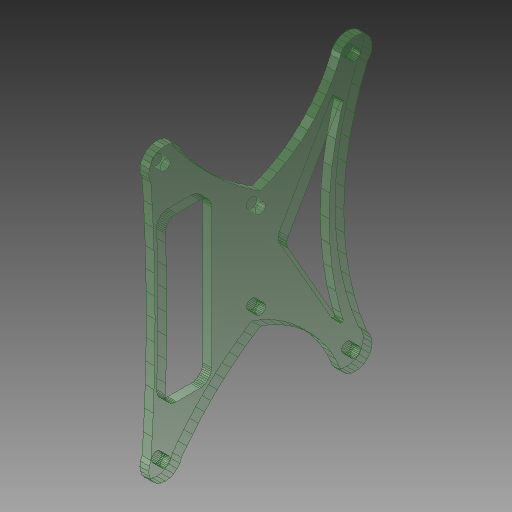
# Autodesk Inventor part: LCD Back
Saved by Autodesk Inventor 2017 (Build 210142000, 142)
## iProperties
Created: 2016-07-27
Part Number: LCD Back
Material: Polycarbonate, Green
Document SubType Name: Modeling
Designer: User
Density: 1.2 g/cm^3
Appearance: Polycarbonate - Clear(2)
Author: User
Autodesk Inventor part; units mm, degrees
ref_plane "YZ Plane" through (0, 0, 0) normal (1, 0, 0) x (0, 1, 0)
ref_plane "XZ Plane" through (0, 0, 0) normal (0, 1, 0) x (-1, 0, 0)
ref_plane "XY Plane" through (0, 0, 0) normal (0, 0, 1) x (1, 0, 0)
sketch "Sketch1" plane through (0, 0, 0) normal (1, 0, 0) x (0, 1, 0)
  line L0 (99.8582, 85.8976) -> (98.9523, 87.0781)
  line L1 (98.9523, 87.0781) -> (97.7718, 87.984)
  line L2 (97.7718, 87.984) -> (96.3971, 88.5535)
  line L3 (96.3971, 88.5535) -> (93.4934, 89.8678)
  line L4 (93.4934, 89.8678) -> (90.6898, 91.384)
  line L5 (90.6898, 91.384) -> (88.0005, 93.0948)
  line L6 (88.0005, 93.0948) -> (85.4388, 94.9914)
  line L7 (85.4388, 94.9914) -> (83.0176, 97.0643)
  line L8 (83.0176, 97.0643) -> (80.7493, 99.3035)
  line L9 (80.7493, 99.3035) -> (78.645, 101.6974)
  line L10 (78.645, 101.6974) -> (76.7151, 104.2342)
  line L11 (76.7151, 104.2342) -> (74.9695, 106.901)
  line L12 (74.9695, 106.901) -> (73.4169, 109.6846)
  line L13 (73.4169, 109.6846) -> (72.0648, 112.571)
  line L14 (72.0648, 112.571) -> (70.9203, 115.5457)
  line L15 (70.9203, 115.5457) -> (72.6238, 118.1505)
  line L16 (72.6238, 118.1505) -> (74.4103, 120.699)
  line L17 (74.4103, 120.699) -> (76.2779, 123.1886)
  line L18 (76.2779, 123.1886) -> (78.2249, 125.6168)
  line L19 (78.2249, 125.6168) -> (80.2491, 127.9809)
  line L20 (80.2491, 127.9809) -> (82.3484, 130.2786)
  line L21 (82.3484, 130.2786) -> (84.5207, 132.5074)
  line L22 (84.5207, 132.5074) -> (86.7637, 134.6651)
  line L23 (86.7637, 134.6651) -> (89.075, 136.7494)
  line L24 (89.075, 136.7494) -> (91.4523, 138.7582)
  line L25 (91.4523, 138.7582) -> (93.8931, 140.6893)
  line L26 (93.8931, 140.6893) -> (96.394, 142.5437)
  line L27 (96.394, 142.5437) -> (97.7687, 143.1132)
  line L28 (97.7687, 143.1132) -> (98.9492, 144.0191)
  line L29 (98.9492, 144.0191) -> (99.8551, 145.1995)
  line L30 (99.8551, 145.1995) -> (100.4246, 146.5743)
  line L31 (100.4246, 146.5743) -> (100.6188, 148.0495)
  line L32 (100.6188, 148.0495) -> (100.4246, 149.5241)
  line L33 (100.4246, 149.5241) -> (99.8552, 150.8989)
  line L34 (99.8552, 150.8989) -> (98.9493, 152.0793)
  line L35 (98.9493, 152.0793) -> (97.7688, 152.9852)
  line L36 (97.7688, 152.9852) -> (96.3941, 153.5547)
  line L37 (96.3941, 153.5547) -> (94.9188, 153.7489)
  line L38 (94.9188, 153.7489) -> (93.4436, 153.5547)
  line L39 (93.4436, 153.5547) -> (93.2768, 153.4856)
  line L40 (93.2768, 153.4856) -> (92.0689, 152.9852)
  line L41 (92.0689, 152.9852) -> (85.2186, 152.5575)
  line L42 (85.2186, 152.5575) -> (78.3639, 152.2075)
  line L43 (78.3639, 152.2075) -> (71.5057, 151.9352)
  line L44 (71.5057, 151.9352) -> (64.6449, 151.7407)
  line L45 (64.6449, 151.7407) -> (57.7823, 151.624)
  line L46 (57.7823, 151.624) -> (50.9188, 151.5851)
  line L47 (50.9188, 151.5851) -> (44.0554, 151.624)
  line L48 (44.0554, 151.624) -> (37.1928, 151.7407)
  line L49 (37.1928, 151.7407) -> (30.332, 151.9352)
  line L50 (30.332, 151.9352) -> (23.4738, 152.2077)
  line L51 (23.4738, 152.2077) -> (16.6191, 152.5579)
  line L52 (16.6191, 152.5579) -> (9.7689, 152.9858)
  line L53 (9.7689, 152.9858) -> (8.3942, 153.5553)
  line L54 (8.3942, 153.5553) -> (6.9189, 153.7495)
  line L55 (6.9189, 153.7495) -> (5.4436, 153.5553)
  line L56 (5.4436, 153.5553) -> (4.0689, 152.9858)
  line L57 (4.0689, 152.9858) -> (2.8885, 152.0799)
  line L58 (2.8885, 152.0799) -> (1.9826, 150.8995)
  line L59 (1.9826, 150.8995) -> (1.4131, 149.5248)
  line L60 (1.4131, 149.5248) -> (1.2189, 148.0495)
  line L61 (1.2189, 148.0495) -> (1.4131, 146.5742)
  line L62 (1.4131, 146.5742) -> (1.9825, 145.1995)
  line L63 (1.9825, 145.1995) -> (2.8884, 144.019)
  line L64 (2.8884, 144.019) -> (4.0689, 143.1131)
  line L65 (4.0689, 143.1131) -> (5.4436, 142.5436)
  line L66 (5.4436, 142.5436) -> (7.9456, 140.6925)
  line L67 (7.9456, 140.6925) -> (10.3866, 138.7617)
  line L68 (10.3866, 138.7617) -> (12.7641, 136.7533)
  line L69 (12.7641, 136.7533) -> (15.0757, 134.6693)
  line L70 (15.0757, 134.6693) -> (17.3189, 132.5118)
  line L71 (17.3189, 132.5118) -> (19.4915, 130.2833)
  line L72 (19.4915, 130.2833) -> (21.5911, 127.9858)
  line L73 (21.5911, 127.9858) -> (23.6155, 125.6219)
  line L74 (23.6155, 125.6219) -> (25.5628, 123.194)
  line L75 (25.5628, 123.194) -> (27.4308, 120.7046)
  line L76 (27.4308, 120.7046) -> (29.2176, 118.1563)
  line L77 (29.2176, 118.1563) -> (30.9214, 115.5518)
  line L78 (30.9214, 115.5518) -> (29.7772, 112.5769)
  line L79 (29.7772, 112.5769) -> (28.4256, 109.6903)
  line L80 (28.4256, 109.6903) -> (26.8732, 106.9066)
  line L81 (26.8732, 106.9066) -> (25.1279, 104.2395)
  line L82 (25.1279, 104.2395) -> (23.1984, 101.7025)
  line L83 (23.1984, 101.7025) -> (21.0943, 99.3084)
  line L84 (21.0943, 99.3084) -> (18.8263, 97.0689)
  line L85 (18.8263, 97.0689) -> (16.4054, 94.9957)
  line L86 (16.4054, 94.9957) -> (13.8439, 93.0988)
  line L87 (13.8439, 93.0988) -> (11.1548, 91.3877)
  line L88 (11.1548, 91.3877) -> (8.3514, 89.8711)
  line L89 (8.3514, 89.8711) -> (5.4478, 88.5565)
  line L90 (5.4478, 88.5565) -> (4.0731, 87.987)
  line L91 (4.0731, 87.987) -> (2.8926, 87.0811)
  line L92 (2.8926, 87.0811) -> (1.9867, 85.9006)
  line L93 (1.9867, 85.9006) -> (1.4172, 84.5259)
  line L94 (1.4172, 84.5259) -> (1.223, 83.0507)
  line L95 (1.223, 83.0507) -> (1.4172, 81.5754)
  line L96 (1.4172, 81.5754) -> (1.9867, 80.2007)
  line L97 (1.9867, 80.2007) -> (2.8926, 79.0202)
  line L98 (2.8926, 79.0202) -> (4.0731, 78.1143)
  line L99 (4.0731, 78.1143) -> (5.4478, 77.5448)
  line L100 (5.4478, 77.5448) -> (6.923, 77.3506)
  line L101 (6.923, 77.3506) -> (8.3983, 77.5448)
  line L102 (8.3983, 77.5448) -> (9.773, 78.1143)
  line L103 (9.773, 78.1143) -> (11.0884, 79.0713)
  line L104 (11.0884, 79.0713) -> (17.3468, 81.4425)
  line L105 (17.3468, 81.4425) -> (22.6145, 83.0508)
  line L106 (22.6145, 83.0508) -> (23.8857, 83.4389)
  line L107 (23.8857, 83.4389) -> (30.5418, 85.0007)
  line L108 (30.5418, 85.0007) -> (37.2863, 86.1211)
  line L109 (37.2863, 86.1211) -> (44.0898, 86.7953)
  line L110 (44.0898, 86.7953) -> (50.9229, 87.0204)
  line L111 (50.9229, 87.0204) -> (57.7561, 86.7954)
  line L112 (57.7561, 86.7954) -> (64.5596, 86.1212)
  line L113 (64.5596, 86.1212) -> (71.3041, 85.0009)
  line L114 (71.3041, 85.0009) -> (77.9602, 83.4392)
  line L115 (77.9602, 83.4392) -> (79.2314, 83.0511)
  line L116 (79.2314, 83.0511) -> (84.4991, 81.4428)
  line L117 (84.4991, 81.4428) -> (90.7575, 79.0716)
  line L118 (90.7575, 79.0716) -> (90.8924, 79.0205)
  line L119 (90.8924, 79.0205) -> (92.0729, 78.1146)
  line L120 (92.0729, 78.1146) -> (93.4476, 77.5451)
  line L121 (93.4476, 77.5451) -> (94.9229, 77.3509)
  line L122 (94.9229, 77.3509) -> (96.3981, 77.5451)
  line L123 (96.3981, 77.5451) -> (97.7729, 78.1146)
  line L124 (97.7729, 78.1146) -> (98.9533, 79.0205)
  line L125 (98.9533, 79.0205) -> (99.858, 80.1993)
  line L126 (99.858, 80.1993) -> (100.4275, 81.574)
  line L127 (100.4275, 81.574) -> (100.6217, 83.0492)
  line L128 (100.6217, 83.0492) -> (100.4277, 84.5229)
  line L129 (100.4277, 84.5229) -> (99.8582, 85.8976)
  line L130 (96.5664, 148.4895) -> (96.3966, 148.8995)
  line L131 (96.3966, 148.8995) -> (96.1264, 149.2515)
  line L132 (96.1264, 149.2515) -> (95.7743, 149.5217)
  line L133 (95.7743, 149.5217) -> (95.3643, 149.6915)
  line L134 (95.3643, 149.6915) -> (94.9243, 149.7495)
  line L135 (94.9243, 149.7495) -> (94.4843, 149.6916)
  line L136 (94.4843, 149.6916) -> (94.0743, 149.5217)
  line L137 (94.0743, 149.5217) -> (93.7223, 149.2515)
  line L138 (93.7223, 149.2515) -> (93.4521, 148.8995)
  line L139 (93.4521, 148.8995) -> (93.2822, 148.4895)
  line L140 (93.2822, 148.4895) -> (93.2243, 148.0495)
  line L141 (93.2243, 148.0495) -> (93.2822, 147.6095)
  line L142 (93.2822, 147.6095) -> (93.3265, 147.5026)
  line L143 (93.3265, 147.5026) -> (93.4521, 147.1995)
  line L144 (93.4521, 147.1995) -> (93.7223, 146.8474)
  line L145 (93.7223, 146.8474) -> (94.0744, 146.5772)
  line L146 (94.0744, 146.5772) -> (94.4843, 146.4074)
  line L147 (94.4843, 146.4074) -> (94.9243, 146.3494)
  line L148 (94.9243, 146.3494) -> (95.3643, 146.4074)
  line L149 (95.3643, 146.4074) -> (95.7743, 146.5772)
  line L150 (95.7743, 146.5772) -> (96.1264, 146.8474)
  line L151 (96.1264, 146.8474) -> (96.3966, 147.1995)
  line L152 (96.3966, 147.1995) -> (96.5664, 147.6094)
  line L153 (96.5664, 147.6094) -> (96.6243, 148.0494)
  line L154 (96.6243, 148.0494) -> (96.5664, 148.4895)
  line L155 (78.5162, 144.7192) -> (78.4132, 145.2247)
  line L156 (78.4132, 145.2247) -> (78.2435, 145.7119)
  line L157 (78.2435, 145.7119) -> (78.0103, 146.1721)
  line L158 (78.0103, 146.1721) -> (77.7176, 146.597)
  line L159 (77.7176, 146.597) -> (77.3708, 146.9789)
  line L160 (77.3708, 146.9789) -> (76.9761, 147.3111)
  line L161 (76.9761, 147.3111) -> (76.5405, 147.5875)
  line L162 (76.5405, 147.5875) -> (76.0719, 147.8033)
  line L163 (76.0719, 147.8033) -> (75.5786, 147.9545)
  line L164 (75.5786, 147.9545) -> (75.0696, 148.0384)
  line L165 (75.0696, 148.0384) -> (74.5539, 148.0536)
  line L166 (74.5539, 148.0536) -> (71.6473, 147.9381)
  line L167 (71.6473, 147.9381) -> (64.7411, 147.7424)
  line L168 (64.7411, 147.7424) -> (57.8332, 147.6249)
  line L169 (57.8332, 147.6249) -> (50.9243, 147.5857)
  line L170 (50.9243, 147.5857) -> (44.0155, 147.6249)
  line L171 (44.0155, 147.6249) -> (37.1076, 147.7424)
  line L172 (37.1076, 147.7424) -> (30.2014, 147.9381)
  line L173 (30.2014, 147.9381) -> (26.8482, 148.0682)
  line L174 (26.8482, 148.0682) -> (26.3322, 148.0522)
  line L175 (26.3322, 148.0522) -> (25.8229, 147.9675)
  line L176 (25.8229, 147.9675) -> (25.3295, 147.8156)
  line L177 (25.3295, 147.8156) -> (24.8608, 147.5991)
  line L178 (24.8608, 147.5991) -> (24.4251, 147.322)
  line L179 (24.4251, 147.322) -> (24.0305, 146.9893)
  line L180 (24.0305, 146.9893) -> (23.6837, 146.6068)
  line L181 (23.6837, 146.6068) -> (23.3911, 146.1814)
  line L182 (23.3911, 146.1814) -> (23.1579, 145.7208)
  line L183 (23.1579, 145.7208) -> (22.9883, 145.2332)
  line L184 (22.9883, 145.2332) -> (22.8853, 144.7273)
  line L185 (22.8853, 144.7273) -> (22.8508, 144.2122)
  line L186 (22.8508, 144.2122) -> (22.8508, 136.3352)
  line L187 (22.8508, 136.3352) -> (22.8847, 135.8071)
  line L188 (22.8847, 135.8071) -> (22.986, 135.2877)
  line L189 (22.986, 135.2877) -> (23.1529, 134.7855)
  line L190 (23.1529, 134.7855) -> (23.3828, 134.3089)
  line L191 (23.3828, 134.3089) -> (23.6717, 133.8656)
  line L192 (23.6717, 133.8656) -> (24.0151, 133.463)
  line L193 (24.0151, 133.463) -> (24.4072, 133.1076)
  line L194 (24.4072, 133.1076) -> (24.8415, 132.8053)
  line L195 (24.8415, 132.8053) -> (25.311, 132.5611)
  line L196 (25.311, 132.5611) -> (25.8079, 132.3791)
  line L197 (25.8079, 132.3791) -> (26.324, 132.2621)
  line L198 (26.324, 132.2621) -> (26.8508, 132.2122)
  line L199 (26.8508, 132.2122) -> (74.5507, 132.2122)
  line L200 (74.5507, 132.2122) -> (75.0729, 132.2464)
  line L201 (75.0729, 132.2464) -> (75.586, 132.3485)
  line L202 (75.586, 132.3485) -> (76.0815, 132.5167)
  line L203 (76.0815, 132.5167) -> (76.5507, 132.7482)
  line L204 (76.5507, 132.7482) -> (76.9858, 133.0389)
  line L205 (76.9858, 133.0389) -> (77.3791, 133.3839)
  line L206 (77.3791, 133.3839) -> (77.7242, 133.7772)
  line L207 (77.7242, 133.7772) -> (78.0149, 134.2122)
  line L208 (78.0149, 134.2122) -> (78.2463, 134.6815)
  line L209 (78.2463, 134.6815) -> (78.4146, 135.177)
  line L210 (78.4146, 135.177) -> (78.5167, 135.6901)
  line L211 (78.5167, 135.6901) -> (78.5508, 136.2122)
  line L212 (78.5508, 136.2122) -> (78.5508, 144.2045)
  line L213 (78.5508, 144.2045) -> (78.5162, 144.7192)
  line L214 (67.5664, 115.9894) -> (67.3966, 116.3994)
  line L215 (67.3966, 116.3994) -> (67.1264, 116.7515)
  line L216 (67.1264, 116.7515) -> (66.7744, 117.0217)
  line L217 (66.7744, 117.0217) -> (66.3643, 117.1915)
  line L218 (66.3643, 117.1915) -> (65.9244, 117.2494)
  line L219 (65.9244, 117.2494) -> (65.4842, 117.1915)
  line L220 (65.4842, 117.1915) -> (65.0744, 117.0217)
  line L221 (65.0744, 117.0217) -> (64.7223, 116.7515)
  line L222 (64.7223, 116.7515) -> (64.4521, 116.3995)
  line L223 (64.4521, 116.3995) -> (64.2823, 115.9895)
  line L224 (64.2823, 115.9895) -> (64.2244, 115.5495)
  line L225 (64.2244, 115.5495) -> (64.2823, 115.1095)
  line L226 (64.2823, 115.1095) -> (64.4521, 114.6995)
  line L227 (64.4521, 114.6995) -> (64.7223, 114.3474)
  line L228 (64.7223, 114.3474) -> (65.0744, 114.0772)
  line L229 (65.0744, 114.0772) -> (65.4844, 113.9074)
  line L230 (65.4844, 113.9074) -> (65.9243, 113.8495)
  line L231 (65.9243, 113.8495) -> (66.3644, 113.9074)
  line L232 (66.3644, 113.9074) -> (66.7744, 114.0772)
  line L233 (66.7744, 114.0772) -> (67.1265, 114.3474)
  line L234 (67.1265, 114.3474) -> (67.3967, 114.6995)
  line L235 (67.3967, 114.6995) -> (67.5665, 115.1095)
  line L236 (67.5665, 115.1095) -> (67.6244, 115.5493)
  line L237 (67.6244, 115.5493) -> (67.5664, 115.9894)
  line L238 (96.5664, 83.4894) -> (96.3966, 83.8994)
  line L239 (96.3966, 83.8994) -> (96.1264, 84.2515)
  line L240 (96.1264, 84.2515) -> (95.7744, 84.5217)
  line L241 (95.7744, 84.5217) -> (95.3644, 84.6915)
  line L242 (95.3644, 84.6915) -> (94.9243, 84.7494)
  line L243 (94.9243, 84.7494) -> (94.4844, 84.6915)
  line L244 (94.4844, 84.6915) -> (94.0744, 84.5217)
  line L245 (94.0744, 84.5217) -> (93.7223, 84.2515)
  line L246 (93.7223, 84.2515) -> (93.4521, 83.8994)
  line L247 (93.4521, 83.8994) -> (93.3525, 83.6589)
  line L248 (93.3525, 83.6589) -> (93.2822, 83.4895)
  line L249 (93.2822, 83.4895) -> (93.2243, 83.0495)
  line L250 (93.2243, 83.0495) -> (93.2822, 82.6095)
  line L251 (93.2822, 82.6095) -> (93.4521, 82.1995)
  line L252 (93.4521, 82.1995) -> (93.7223, 81.8474)
  line L253 (93.7223, 81.8474) -> (94.0743, 81.5772)
  line L254 (94.0743, 81.5772) -> (94.4843, 81.4074)
  line L255 (94.4843, 81.4074) -> (94.9243, 81.3495)
  line L256 (94.9243, 81.3495) -> (95.3644, 81.4074)
  line L257 (95.3644, 81.4074) -> (95.7743, 81.5772)
  line L258 (95.7743, 81.5772) -> (96.1264, 81.8474)
  line L259 (96.1264, 81.8474) -> (96.3966, 82.1995)
  line L260 (96.3966, 82.1995) -> (96.5664, 82.6095)
  line L261 (96.5664, 82.6095) -> (96.6244, 83.0495)
  line L262 (96.6244, 83.0495) -> (96.5664, 83.4894)
  line L263 (83.7845, 88.0859) -> (83.5631, 88.263)
  line L264 (83.5631, 88.263) -> (52.651, 106.0557)
  line L265 (52.651, 106.0557) -> (52.1053, 106.3095)
  line L266 (52.1053, 106.3095) -> (51.5239, 106.4649)
  line L267 (51.5239, 106.4649) -> (51.2253, 106.5041)
  line L268 (51.2253, 106.5041) -> (50.6235, 106.5041)
  line L269 (50.6235, 106.5041) -> (50.3248, 106.4649)
  line L270 (50.3248, 106.4649) -> (49.7434, 106.3096)
  line L271 (49.7434, 106.3096) -> (49.1977, 106.0559)
  line L272 (49.1977, 106.0559) -> (18.2833, 88.2672)
  line L273 (18.2833, 88.2672) -> (18.0618, 88.0902)
  line L274 (18.0618, 88.0902) -> (17.9585, 87.8262)
  line L275 (17.9585, 87.8262) -> (17.9613, 87.6833)
  line L276 (17.9613, 87.6833) -> (18.0749, 87.4235)
  line L277 (18.0749, 87.4235) -> (18.178, 87.3245)
  line L278 (18.178, 87.3245) -> (18.442, 87.2211)
  line L279 (18.442, 87.2211) -> (18.7223, 87.2637)
  line L280 (18.7223, 87.2637) -> (21.1418, 88.0191)
  line L281 (21.1418, 88.0191) -> (28.4688, 89.7764)
  line L282 (28.4688, 89.7764) -> (35.8974, 91.0373)
  line L283 (35.8974, 91.0373) -> (43.3938, 91.7961)
  line L284 (43.3938, 91.7961) -> (50.9243, 92.0495)
  line L285 (50.9243, 92.0495) -> (58.4549, 91.7961)
  line L286 (58.4549, 91.7961) -> (65.9513, 91.0373)
  line L287 (65.9513, 91.0373) -> (73.3799, 89.7764)
  line L288 (73.3799, 89.7764) -> (80.7069, 88.0191)
  line L289 (80.7069, 88.0191) -> (83.1264, 87.2637)
  line L290 (83.1264, 87.2637) -> (83.2638, 87.2239)
  line L291 (83.2638, 87.2239) -> (83.5455, 87.2554)
  line L292 (83.5455, 87.2554) -> (83.7738, 87.4235)
  line L293 (83.7738, 87.4235) -> (83.8874, 87.6833)
  line L294 (83.8874, 87.6833) -> (83.8878, 87.8219)
  line L295 (83.8878, 87.8219) -> (83.7845, 88.0859)
  line L296 (8.5664, 83.4895) -> (8.4962, 83.6589)
  line L297 (8.4962, 83.6589) -> (8.3966, 83.8995)
  line L298 (8.3966, 83.8995) -> (8.1264, 84.2515)
  line L299 (8.1264, 84.2515) -> (7.7744, 84.5217)
  line L300 (7.7744, 84.5217) -> (7.3644, 84.6915)
  line L301 (7.3644, 84.6915) -> (6.9243, 84.7495)
  line L302 (6.9243, 84.7495) -> (6.4844, 84.6916)
  line L303 (6.4844, 84.6916) -> (6.0743, 84.5217)
  line L304 (6.0743, 84.5217) -> (5.7223, 84.2515)
  line L305 (5.7223, 84.2515) -> (5.4521, 83.8995)
  line L306 (5.4521, 83.8995) -> (5.2823, 83.4895)
  line L307 (5.2823, 83.4895) -> (5.2243, 83.0495)
  line L308 (5.2243, 83.0495) -> (5.2823, 82.6095)
  line L309 (5.2823, 82.6095) -> (5.4521, 82.1995)
  line L310 (5.4521, 82.1995) -> (5.7223, 81.8474)
  line L311 (5.7223, 81.8474) -> (6.0743, 81.5772)
  line L312 (6.0743, 81.5772) -> (6.4843, 81.4074)
  line L313 (6.4843, 81.4074) -> (6.9243, 81.3495)
  line L314 (6.9243, 81.3495) -> (7.3643, 81.4074)
  line L315 (7.3643, 81.4074) -> (7.7743, 81.5772)
  line L316 (7.7743, 81.5772) -> (8.1264, 81.8474)
  line L317 (8.1264, 81.8474) -> (8.3966, 82.1994)
  line L318 (8.3966, 82.1994) -> (8.5664, 82.6095)
  line L319 (8.5664, 82.6095) -> (8.6244, 83.0495)
  line L320 (8.6244, 83.0495) -> (8.5664, 83.4895)
  line L321 (8.5664, 148.4895) -> (8.3966, 148.8995)
  line L322 (8.3966, 148.8995) -> (8.1264, 149.2515)
  line L323 (8.1264, 149.2515) -> (7.7744, 149.5217)
  line L324 (7.7744, 149.5217) -> (7.3644, 149.6916)
  line L325 (7.3644, 149.6916) -> (6.9243, 149.7495)
  line L326 (6.9243, 149.7495) -> (6.4843, 149.6916)
  line L327 (6.4843, 149.6916) -> (6.0743, 149.5217)
  line L328 (6.0743, 149.5217) -> (5.7223, 149.2515)
  line L329 (5.7223, 149.2515) -> (5.4521, 148.8995)
  line L330 (5.4521, 148.8995) -> (5.2823, 148.4895)
  line L331 (5.2823, 148.4895) -> (5.2243, 148.0495)
  line L332 (5.2243, 148.0495) -> (5.2823, 147.6095)
  line L333 (5.2823, 147.6095) -> (5.4521, 147.1995)
  line L334 (5.4521, 147.1995) -> (5.7223, 146.8474)
  line L335 (5.7223, 146.8474) -> (6.0744, 146.5772)
  line L336 (6.0744, 146.5772) -> (6.4844, 146.4074)
  line L337 (6.4844, 146.4074) -> (6.9243, 146.3495)
  line L338 (6.9243, 146.3495) -> (7.3644, 146.4074)
  line L339 (7.3644, 146.4074) -> (7.7743, 146.5772)
  line L340 (7.7743, 146.5772) -> (8.1264, 146.8474)
  line L341 (8.1264, 146.8474) -> (8.3966, 147.1995)
  line L342 (8.3966, 147.1995) -> (8.5222, 147.5026)
  line L343 (8.5222, 147.5026) -> (8.5664, 147.6094)
  line L344 (8.5664, 147.6094) -> (8.6244, 148.0495)
  line L345 (8.6244, 148.0495) -> (8.5664, 148.4895)
  line L346 (37.5665, 115.9894) -> (37.3966, 116.3994)
  line L347 (37.3966, 116.3994) -> (37.1264, 116.7515)
  line L348 (37.1264, 116.7515) -> (36.7744, 117.0217)
  line L349 (36.7744, 117.0217) -> (36.3644, 117.1915)
  line L350 (36.3644, 117.1915) -> (35.9244, 117.2494)
  line L351 (35.9244, 117.2494) -> (35.4843, 117.1915)
  line L352 (35.4843, 117.1915) -> (35.0744, 117.0217)
  line L353 (35.0744, 117.0217) -> (34.7223, 116.7515)
  line L354 (34.7223, 116.7515) -> (34.4521, 116.3995)
  line L355 (34.4521, 116.3995) -> (34.2823, 115.9895)
  line L356 (34.2823, 115.9895) -> (34.2244, 115.5495)
  line L357 (34.2244, 115.5495) -> (34.2823, 115.1095)
  line L358 (34.2823, 115.1095) -> (34.4521, 114.6995)
  line L359 (34.4521, 114.6995) -> (34.7223, 114.3474)
  line L360 (34.7223, 114.3474) -> (35.0744, 114.0772)
  line L361 (35.0744, 114.0772) -> (35.4844, 113.9074)
  line L362 (35.4844, 113.9074) -> (35.9244, 113.8495)
  line L363 (35.9244, 113.8495) -> (36.3644, 113.9074)
  line L364 (36.3644, 113.9074) -> (36.7744, 114.0772)
  line L365 (36.7744, 114.0772) -> (37.1264, 114.3474)
  line L366 (37.1264, 114.3474) -> (37.3966, 114.6995)
  line L367 (37.3966, 114.6995) -> (37.5665, 115.1095)
  line L368 (37.5665, 115.1095) -> (37.6244, 115.5494)
  line L369 (37.6244, 115.5494) -> (37.5665, 115.9894)
  point P0 (0, 0)
  constraints: 740 end point, 103 parallel, 101 perpendicular, 3 collinear
extrude "Extrusion1" add sketch "Sketch1" along normal blind 3
sketch "Sketch2" plane through (0, 0, 0) normal (-1, 0, 0) x (0, 0, 1)
  line L0 (149.6916, 94.4843) -> (149.7495, 94.9243) projected
  line L1 (146.3494, 94.9243) -> (146.4074, 94.4843) projected
  line L2 (149.7495, 94.9243) -> (146.3494, 94.9243)
  circle A0 centre (148.0495, 94.9243) radius 1.7
  point P0 (0, 0)
  dimension "d2" = 3.4
  constraints: 2 end point, 1 centre point, 1 coincident, 1 midpoint
  measures "d2" diameter of A0
extrude "Extrusion2" cut sketch "Sketch2" against normal through all
sketch "Sketch3" plane through (0, 0, 0) normal (-1, 0, 0) x (0, 0, 1)
  line L0 (117.1915, 66.3643) -> (117.2494, 65.9244) projected
  line L1 (117.2494, 65.9244) -> (113.8491, 65.9244)
  circle A0 centre (115.5493, 65.9244) radius 1.75
  point P0 (0, 0)
  dimension "d5" = 3.5
  constraints: 2 end point, 1 centre point, 1 horizontal, 1 midpoint
  measures "d5" diameter of A0
extrude "Extrusion3" cut sketch "Sketch3" against normal through all
body "Solid1"
